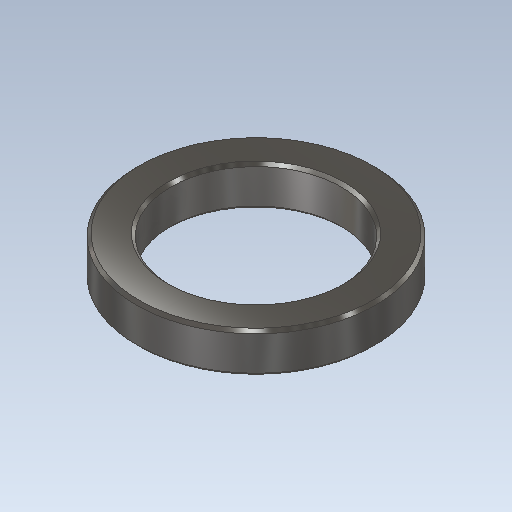
# Autodesk Inventor part: bearing_30x42x7
Saved by Autodesk Inventor 2020 (Build 240168000, 168)
## iProperties
Created: 2019-11-01
Part Number: bearing_30x42x7
Material: Generic
Document SubType Name: Modeling
Designer: xhsxb
Density: 1 g/cm^3
Appearance: Steel - Polished
Mass: 4.69354 g
Surface Area: 28.0803 cm^2
Volume: 4.69354 cm^3
Author: xhsxb
Autodesk Inventor part; units mm, degrees
ref_plane "YZ Plane" through (0, 0, 0) normal (1, 0, 0) x (0, 1, 0)
ref_plane "XZ Plane" through (0, 0, 0) normal (0, 1, 0) x (-1, 0, 0)
ref_plane "XY Plane" through (0, 0, 0) normal (0, 0, 1) x (1, 0, 0)
sketch "Sketch1" plane through (0, 0, 0) normal (0, 1, 0) x (-1, 0, 0)
  circle A0 centre (0, 0) radius 15
  circle A1 centre (0, 0) radius 21
  dimension "d0" = 30
  dimension "d1" = 42
  constraints: 2 centre point, 2 coincident
  measures "d0" diameter of A0
  measures "d1" diameter of A1
extrude "Extrusion1" add sketch "Sketch1" along normal blind 7
chamfer "Chamfer1" distance 0.5 angle 45 4 edges at (21, 7, 0) (21, 0, 0) (15, 0, 0) (15, 7, 0)
body "Solid1"
